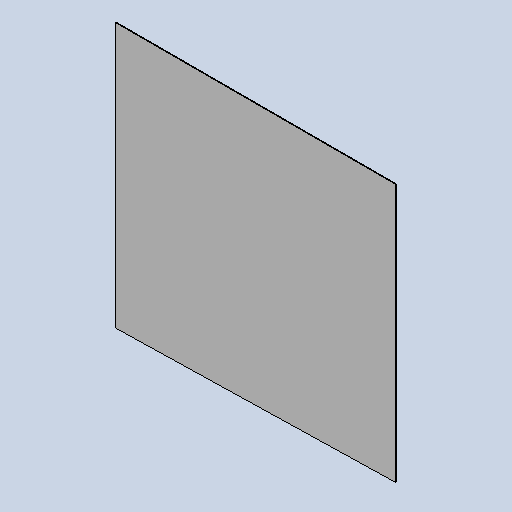
# Autodesk Inventor part: GBK 3111 shield 1
Saved by Autodesk Inventor 2026.2 (Build 302298010, 298A)
## iProperties
Created: 2026-04-17
Part Number: GBK 3111 shield 1
Material: Steel
Document SubType Name: Sheet Metal
Designer: pokla
Stock Number: 3111
Mass: 64187.5 g
Surface Area: 41112.6 cm^2
Volume: 8176.75 cm^3
Density: 7.85 g/cm^3
Flat Pattern Width: 139.8 cm
Flat Pattern Length: 148 cm
Flat Pattern Area: 20690.4 cm^2
Sheet Metal Rule: Default_mm
Sheet Metal Width: 1398,000 мм
Sheet Metal Length: 1480,000 мм
Sheet Metal Area: 2069040,000 мм^2
Appearance: Default
Author: admin
Autodesk Inventor part; units mm, degrees
ref_plane "YZ Plane" through (0, 0, 0) normal (1, 0, 0) x (0, 1, 0)
ref_plane "XZ Plane" through (0, 0, 0) normal (0, 1, 0) x (-1, 0, 0)
ref_plane "XY Plane" through (0, 0, 0) normal (0, 0, 1) x (1, 0, 0)
sketch "Sketch1" plane through (0, 0, 0) normal (0, 0, 1) x (1, 0, 0)
  line L0 (740, -745) -> (-740, -745)
  line L1 (-740, -745) -> (-740, 745)
  line L2 (-740, 745) -> (740, 745)
  line L3 (740, 745) -> (740, -745)
  line L4 (740, -745) -> (-740, 745) construction
  line L5 (-740, -745) -> (740, 745) construction
  line L6 (-740, -653) -> (740, -619.4141)
  point P0 (0, 0)
  dimension "d0" = 1480
  dimension "d1" = 1490
  dimension "d3" = 92
  dimension "d4" = 1.3
  measures "d0" distance of L1.end L2.end
  measures "d1" distance of L0.end L1.end
  measures "d3" distance of L0.end L6.start
  measures "d4" angle of L0 L6
extrude "Plate1" add sketch "Sketch1" along normal blind 4 contours L6 L1 L2 L3
sketch "Эскиз4" plane through (0, 0, 0) normal (0, 0, -1) x (-1, 0, 0)
  line L0 (549.4783, -556.3714) -> (549.4783, -1054.5075) construction
  line L1 (549.4783, -1054.5075) -> (509.8511, -1054.5075) construction
  line L2 (509.8511, -1054.5075) -> (509.8511, -556.3714) construction
  line L3 (509.8511, -556.3714) -> (549.4783, -556.3714) construction
  line L4 (669.2463, -492.5) -> (669.2463, -589.5) projected
  line L5 (669.2463, -589.5) -> (665.2463, -589.5) projected
  line L6 (169.3732, -492.5) -> (169.3732, -589.5) projected
  line L7 (169.3732, -589.5) -> (165.3732, -589.5) projected
  line L8 (-330.5, -492.5) -> (-330.5, -589.5) projected
  line L9 (-330.5, -589.5) -> (-334.5, -589.5) projected
  line L10 (669.2463, 715.5) -> (669.2463, 775.5) projected
  line L11 (669.2463, 715.5) -> (665.2463, 715.5) projected
  line L12 (169.3732, 715.5) -> (169.3732, 775.5) projected
  line L13 (169.3732, 715.5) -> (165.3732, 715.5) projected
  line L14 (-330.5, 715.5) -> (-330.5, 775.5) projected
  line L15 (-330.5, 715.5) -> (-334.5, 715.5) projected
  line L16 (709.6246, -489) -> (769.6246, -489) projected
  line L17 (709.6246, -489) -> (709.6246, -485) projected
  line L18 (709.6246, 7.6667) -> (769.6246, 7.6667) projected
  line L19 (709.6246, 7.6667) -> (709.6246, 11.6667) projected
  line L20 (709.6246, 504.3333) -> (769.6246, 504.3333) projected
  line L21 (709.6246, 504.3333) -> (709.6246, 508.3333) projected
  line L22 (-740, -489) -> (-710, -489) projected
  line L23 (-710, -489) -> (-710, -485) projected
  line L24 (-740, 7.6667) -> (-710, 7.6667) projected
  line L25 (-710, 7.6667) -> (-710, 11.6667) projected
  line L26 (-740, 504.3333) -> (-710, 504.3333) projected
  line L27 (-710, 504.3333) -> (-710, 508.3333) projected
  point P0 (0, 0)
  constraints: 2 other
mark "Маркировка3"
equation "\"d0\" = Лист_ширина"
equation "\"d1\" = 0.5 * Лист_длина"
equation "\"d2\" = Thickness"
equation "\"BendRadius\" = Thickness"
equation "\"BendReliefWidth\" = Thickness"
equation "\"BendReliefDepth\" = 0.5 * Thickness"
equation "\"CornerReliefSize\" = 4 * Thickness"
equation "\"MinimumRemnant\" = 2 * Thickness"
equation "\"TransitionRadius\" = BendRadius"
equation "\"JacobiRadiusSize\" = BendRadius"
equation "\"GapSize\" = Thickness"
equation "\"Лист_ширина\" = 1480"
equation "\"Лист_длина\" = 2980"
equation "\"Thickness\" = 4"
body "Solid1"
